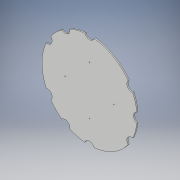
# Autodesk Inventor part: napduoinew
Saved by Autodesk Inventor 2019 (Build 230136000, 136)
## iProperties
Created: 2021-01-20
Part Number: napduoinew
Material: Generic
Document SubType Name: Modeling
Designer: Admin
Density: 1 g/cm^3
Appearance: Default
Author: Admin
Autodesk Inventor part; units mm, degrees
ref_plane "YZ Plane" through (0, 0, 0) normal (1, 0, 0) x (0, 1, 0)
ref_plane "XZ Plane" through (0, 0, 0) normal (0, 1, 0) x (-1, 0, 0)
ref_plane "XY Plane" through (0, 0, 0) normal (0, 0, 1) x (1, 0, 0)
sketch "Sketch1" plane through (0, 0, 0) normal (0, 0, 1) x (1, 0, 0)
  arc A0 (-19.0983, 194.0625) -> (19.0983, 194.0625) centre (0, 200) ccw
  arc A1 (-113.5709, 158.5139) -> (-80.4916, 177.6122) centre (-100, 173.2051) ccw
  arc A2 (-177.6122, 80.4916) -> (-158.5139, 113.5709) centre (-173.2051, 100) ccw
  arc A3 (-194.0625, -19.0983) -> (-194.0625, 19.0983) centre (-200, 0) ccw
  arc A4 (-158.5139, -113.5709) -> (-177.6122, -80.4916) centre (-173.2051, -100) ccw
  arc A5 (-80.4916, -177.6122) -> (-113.5709, -158.5139) centre (-100, -173.2051) ccw
  arc A6 (19.0983, -194.0625) -> (-19.0983, -194.0625) centre (0, -200) ccw
  arc A7 (113.5709, -158.5139) -> (80.4916, -177.6122) centre (100, -173.2051) ccw
  arc A8 (177.6122, -80.4916) -> (158.5139, -113.5709) centre (173.2051, -100) ccw
  arc A9 (194.0625, 19.0983) -> (194.0625, -19.0983) centre (200, 0) ccw
  arc A10 (158.5139, 113.5709) -> (177.6122, 80.4916) centre (173.2051, 100) ccw
  arc A11 (80.4916, 177.6122) -> (113.5709, 158.5139) centre (100, 173.2051) ccw
  arc A12 (-113.5709, 158.5139) -> (-158.5139, 113.5709) centre (0, 0) ccw
  arc A13 (-19.0983, 194.0625) -> (-80.4916, 177.6122) centre (0, 0) ccw
  arc A14 (158.5139, 113.5709) -> (19.0983, 194.0625) centre (0, 0) ccw
  arc A15 (194.0625, 19.0983) -> (177.6122, 80.4916) centre (0, 0) ccw
  arc A16 (177.6122, -80.4916) -> (194.0625, -19.0983) centre (0, 0) ccw
  arc A17 (19.0983, -194.0625) -> (158.5139, -113.5709) centre (0, 0) ccw
  arc A18 (-80.4916, -177.6122) -> (-19.0983, -194.0625) centre (0, 0) ccw
  arc A19 (-177.6122, 80.4916) -> (-177.6122, -80.4916) centre (0, 0) ccw
  arc A20 (-158.5139, -113.5709) -> (-113.5709, -158.5139) centre (0, 0) ccw
  line L0 (0, 0) -> (100, 0) construction
  circle A21 centre (-100, 0) radius 1.5
  circle A22 centre (0, -100) radius 1.5
  circle A23 centre (100, 0) radius 1.5
  circle A24 centre (0, 100) radius 1.5
  dimension "d4" = 40
  dimension "d5" = 360
  dimension "d9" = 3
  dimension "d12" = 360
  constraints: 42 point on circle, 25 centre point, 2 end point, 1 horizontal, 58 other
  measures "d4" diameter of A0
  measures "d9" diameter of A21
extrude "Extrusion1" add sketch "Sketch1" along normal blind 5
body "Solid1"
